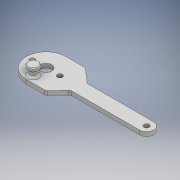
# Autodesk Inventor part: grabber
Saved by Autodesk Inventor 2018.2 (Build 222227000, 227)
## iProperties
Created: 2017-12-31
Part Number: grabber
Material: Generic
Document SubType Name: Modeling
Designer: mzhang
Density: 1 g/cm^3
Appearance: Default
Author: mzhang
Autodesk Inventor part; units mm, degrees
ref_plane "YZ Plane" through (0, 0, 0) normal (1, 0, 0) x (0, 1, 0)
ref_plane "XZ Plane" through (0, 0, 0) normal (0, 1, 0) x (-1, 0, 0)
ref_plane "XY Plane" through (0, 0, 0) normal (0, 0, 1) x (1, 0, 0)
sketch "Sketch1" plane through (0, 0, 0) normal (0, 0, 1) x (1, 0, 0)
  arc A0 (13.0446, 5) -> (13.0446, -5) centre (0, 0) ccw
  circle A1 centre (-9.779, 0) radius 1.8415
  circle A2 centre (9.779, 0) radius 1.8415
  line L0 (76.2, -5) -> (13.0446, -5)
  line L1 (13.0446, -5) -> (13.0446, 5)
  line L2 (13.0446, 5) -> (76.2, 5)
  line L3 (76.2, 5) -> (76.2, -5)
  line L4 (76.2, -5) -> (13.0446, 5) construction
  line L5 (13.0446, -5) -> (76.2, 5) construction
  line L6 (0, 13.97) -> (13.7445, 13.97)
  line L7 (0, -13.97) -> (13.7445, -13.97)
  line L8 (13.7445, -13.97) -> (22.4067, -5)
  line L9 (13.7445, 13.97) -> (24.121, 5)
  line L10 (76.2, -5) -> (76.2, -25)
  line L11 (76.2, -25) -> (66.2, -25)
  circle A3 centre (71.2, -21.0937) radius 2.5
  line L12 (66.2, -25) -> (45.414, -5)
  point P0 (44.6223, 0)
  dimension "d0" = 27.94
  dimension "d1" = 3.683
  dimension "d2" = 3.683
  dimension "d3" = 10
  dimension "d5" = 134
  dimension "d19" = 76.2
  dimension "d36" = 20
  dimension "d37" = 10
  dimension "d38" = 5
  constraints: 26 end point, 4 centre point, 4 point on circle, 3 parallel, 3 point on line, 2 horizontal, 2 midpoint, 2 perpendicular, 1 coincident, 1 tangent, 1 vertical
  measures "d0" diameter of A0
  measures "d1" diameter of A1
  measures "d2" diameter of A2
  measures "d3" distance of L0.end L1.end
  measures "d5" angle of L8 L7
  measures "d19" distance from line of L3 point (0, 0)
  measures "d36" distance of L0.start L10.end
  measures "d37" distance of L10.end L11.end
  measures "d38" diameter of A3
extrude "Extrusion1" add sketch "Sketch1" along normal blind 3
fillet "Fillet1" radius 2 4 edges at (13.7445, -13.97, 1.5) (13.7445, 13.97, 1.5) (24.121, 5, 1.5) (22.4067, -5, 1.5)
extrude "Extrusion11" add sketch "Sketch1" along normal blind 10 contours A3
sketch "Sketch9" plane through (0, 0, 3) normal (0, 0, 1) x (1, 0, 0)
  circle A0 centre (71.2, 0) radius 1.875
  line L0 (76.2, -25) -> (76.2, 5) projected
  point P0 (0, 0)
  dimension "d41" = 3.75
  dimension "d42" = 5
  constraints: 1 centre point
  measures "d41" diameter of A0
  measures "d42" distance from line of L0 A0.centre
extrude "Extrusion12" cut sketch "Sketch9" against normal blind 10
fillet "Fillet3" radius 5 1 edges at (45.414, -5, 1.5)
fillet "Fillet4" radius 10 1 edges at (66.2, -25, 1.5)
chamfer "Chamfer1" distance 2.5 angle 45 1 edges at (76.2, -25, 1.5)
fillet "Fillet5" radius 5 2 edges at (76.2, -22.5, 1.5) (73.7, -25, 1.5)
sketch "Sketch10" plane through (0, 0, 3) normal (0, 0, 1) x (1, 0, 0)
  circle A0 centre (0, -9.1596) radius 2.5
  point P0 (0, 0)
  dimension "d51" = 5
  constraints: 1 centre point
  measures "d51" diameter of A0
extrude "Extrusion13" add sketch "Sketch10" along normal up to surface (7 mm away)
sketch "Sketch11" plane through (0, 0, 3) normal (0, 0, 1) x (1, 0, 0)
  circle A0 centre (0, 0) radius 4
  dimension "d54" = 8
  constraints: 1 centre point, 1 coincident
  measures "d54" diameter of A0
extrude "Extrusion14" cut sketch "Sketch11" against normal up to surface (3 mm away)
fillet "Fillet6" radius 5 1 edges at (76.2, 5, 1.5)
sketch "Sketch12" plane through (71.2, -21.0937, 10) normal (0, 0, 1) x (1, 0, 0)
  circle A0 centre (-71.2, 11.9341) radius 2.5 projected
  circle A1 centre (-71.2, 11.9341) radius 3.75
  circle A2 centre (0, 0) radius 2.5 projected
  circle A3 centre (0, 0) radius 3.75
  point P0 (-71.2, 21.0937)
  dimension "d58" = 7.5
  dimension "d59" = 7.5
  constraints: 2 centre point, 2 coincident
  measures "d58" diameter of A1
  measures "d59" diameter of A3
extrude "Extrusion15" add sketch "Sketch12" against normal blind 2
chamfer "Chamfer2" distance 1.5 angle 45 2 edges at (-2.5, -9.1596, 3) (68.7, -21.0937, 3)
chamfer "Chamfer3" distance 1.25 angle 45 1 edges at (-2.5, -9.1596, 8)
chamfer "Chamfer4" distance 1.25 angle 45 1 edges at (68.7, -21.0937, 8)
chamfer "Chamfer5" distance 0.5 angle 45 2 edges at (67.45, -21.0937, 10) (-3.75, -9.1596, 10)
sketch "Sketch13" plane through (0, 0, 0) normal (0, 0, -1) x (-1, 0, 0)
  line L0 (-76.2, -5) -> (-13.0446, -5) projected
  line L1 (-23.2557, -5) -> (-43.3991, -5) projected
  line L2 (-24.3023, -40.047) -> (-91.4847, -40.047)
  line L3 (-91.4847, -40.047) -> (-91.4847, -5)
  line L4 (-91.4847, -5) -> (-24.3023, -5)
  line L5 (-24.3023, -5) -> (-24.3023, -40.047)
  point P0 (0, 0)
  constraints: 8 end point, 2 parallel, 1 horizontal, 1 perpendicular, 1 point on line
extrude "Extrusion16" cut sketch "Sketch13" against normal blind 10
fillet "Fillet7" radius 5 1 edges at (76.2, -5, 1.5)
body "Solid1"
